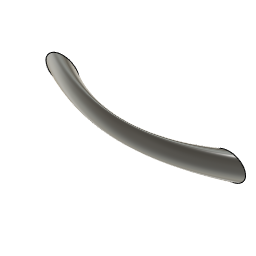
Drawer Cabinet v10 (Autodesk Fusion 360 archive; units mm, degrees)
design "Handle"
Autodesk Fusion 360 part; units mm, degrees
sketch "Sketch1" plane through (0, 0, 0) normal (0, 0, 1) x (1, 0, 0)
  line L0 (0, 0) -> (-88, 0)
  line L1 (0, 0) -> (83, 0)
  ellipse E0 centre (0, 0) end of major axis (75, 0) minor radius 21 (-75, 0) -> (75, 0) ccw
  dimension "d2" = 150
  dimension "d3" = 42
  constraint coincident L0.start L1.start
  measures "d2" distance of E0
sketch "Sketch2" plane through (0, 0, 0) normal (0, 1, 0) x (1, 0, 0)
  ellipse E0 centre (75, 0) end of major axis (90, 0) minor radius 11.5
  line L0 (60, 0) -> (90, 0)
  line L1 (75, -11.5) -> (75, 11.5)
  line L2 (0, -1.75) -> (0, -22.5)
  ellipse E1 centre (-75, 0) end of major axis (-90, 0) minor radius 11.5
  dimension "d4" = 23
  dimension "d5" = 75
  dimension "d6" = 30
  constraint horizontal L0
  constraint coincident E0 L0.start
  constraint coincident E0 L0.end
  constraint coincident E0 L1.start
  constraint coincident E0 L1.end
  constraint horizontal origin E0.centre
  constraint symmetric E0 L2 E1
  measures "d5" distance of E0.centre origin
  measures "d6" distance of E0
sketch "Sketch3" plane through (0, 0, 0) normal (1, 0, 0) x (0, 1, 0)
  ellipse E0 centre (-21, 0) end of major axis (-18, 0) minor radius 9
  line L0 (-24, 0) -> (-18, 0)
  line L1 (-21, -9) -> (-21, 9)
  line L2 (0, 0) -> (-21, 0)
  dimension "d7" = 18
  dimension "d8" = 21
  dimension "d9" = 6
  constraint horizontal L0
  constraint coincident E0 L0.start
  constraint coincident E0 L0.end
  constraint coincident E0 L1.start
  constraint coincident E0 L1.end
  constraint coincident L2.start origin
  constraint coincident E0.centre L2.end
  constraint horizontal L2
  measures "d8" distance of E0.centre L2.start
  measures "d9" distance of E0
loft "Loft1" add profiles "Sketch2", "Sketch3", "Sketch2" section 1 contours E0 L0 L1 | E0 L0 L1 | E0 L0 L1 | E0 L0 L1 section 2 section 3 contours E1
sketch "Sketch4" plane through (0, 0, 0) normal (0, 1, 0) x (-1, 0, 0)
  ellipse E0 centre (-75, 0) end of major axis (-90, 0) minor radius 11.5
  line L0 (0, 1.75) -> (0, 22.5)
  point P0 (-71, 0)
  point P1 (71, 0)
  constraint symmetric P0 L0 P1
hole "Hole1" at (71, 0, 0) direction (0, -1, 0) diameter 5 depth 5 tip angle 118
mirror "Mirror1" about plane through (0, 0, 0) normal (1, 0, 0) of "Hole1"

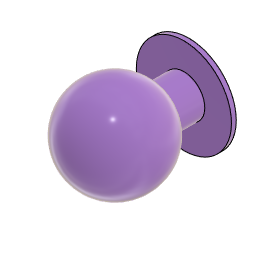
design "Door Handle"
Autodesk Fusion 360 part; units mm, degrees
sketch "Sketch1" plane through (0, 0, 0) normal (1, 0, 0) x (0, 1, 0)
  line L0 (0.5, -0.2195) -> (0.5, 10)
  line L1 (0.5, 10) -> (-0.5, 10)
  line L2 (-6.0151, 4.39) -> (-0.5, 4.39)
  line L3 (0.5, 0.2195) -> (-0.5, -0.2195) construction
  line L4 (-0.5, 0.2195) -> (0.5, -0.2195) construction
  arc A0 (-6.0151, 4.39) -> (-25, 0) centre (-15, 0) ccw
  line L5 (-0.5, 10) -> (-0.5, 4.39)
  line L6 (10, 0) -> (-36.1388, 0)
  line L7 (-0.5, 0.2195) -> (-0.5, -0.2195)
  dimension "d2" = 1
  dimension "d4" = 20
  constraint parallel L0 L5
  constraint horizontal L2
  constraint coincident origin L3
  constraint coincident L0 L3.start
  constraint coincident L3.end L5
  constraint coincident L4.start L5
  constraint collinear L5 L7
  constraint horizontal L6
  constraint coincident L6 A0.end
  measures "d2" distance of L0.end L1.end
  measures "d4" diameter of A0
revolve "Revolve1" add sketch "Sketch1" angle 360 about axis through (0, 10, 0) along (0, -1, 0)
